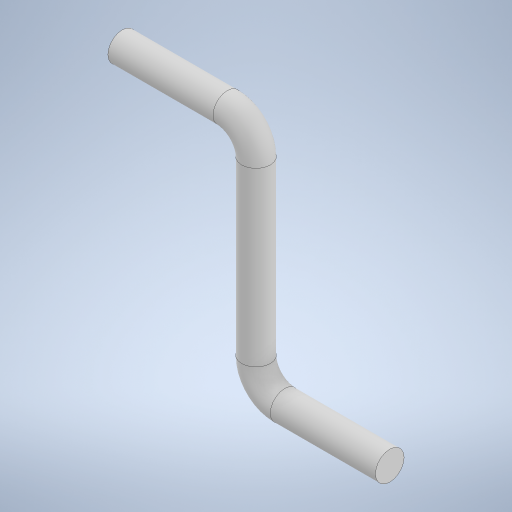
# Autodesk Inventor part: handle
Saved by Autodesk Inventor 2024.2 (Build 282272000, 272)
## iProperties
Created: 2024-05-25
Part Number: handle
Material: Generic
Document SubType Name: Modeling
Designer: user
Density: 1 g/cm^3
Appearance: Default
Author: user
Autodesk Inventor part; units mm, degrees
ref_plane "YZ Plane" through (0, 0, 0) normal (1, 0, 0) x (0, 1, 0)
ref_plane "XZ Plane" through (0, 0, 0) normal (0, 1, 0) x (-1, 0, 0)
ref_plane "XY Plane" through (0, 0, 0) normal (0, 0, 1) x (1, 0, 0)
sketch "Sketch2" plane through (0, 0, 0) normal (0, 0, 1) x (1, 0, 0)
  line L0 (0, 0) -> (-44, 0)
  line L1 (-56, 12) -> (-56, 84)
  line L2 (-68, 96) -> (-112, 96)
  arc A0 (-56, 84) -> (-68, 96) centre (-68, 84) ccw
  arc A1 (-56, 12) -> (-44, 0) centre (-44, 12) ccw
  point P0 (-56, 0)
  point P1 (-56, 96)
  dimension "d0" = 56
  dimension "d1" = 96
  dimension "d2" = 56
  dimension "d3" = 12
  constraints: 6 end point, 4 point on circle, 4 point on line, 4 tangent, 2 centre point, 2 perpendicular, 1 equal radius, 1 horizontal
  measures "d0" distance of L0.start point (-56, 0)
  measures "d1" distance of point (-56, 0) point (-56, 96)
  measures "d2" distance of point (-56, 96) L2.end
  measures "d3" radius of A0
sketch "Sketch3" plane through (0, 0, 0) normal (1, 0, 0) x (0, 1, 0)
  circle A0 centre (0, 0) radius 6
  dimension "d4" = 12
  constraints: 1 centre point, 1 coincident
  measures "d4" diameter of A0
sweep "Sweep1" add profiles "Sketch3" path "Sketch2"
body "Solid1"
